TM Front Holder (Autodesk Fusion 360 design; units mm, degrees)
Autodesk Fusion 360 part; units mm, degrees
sketch "Sketch1" plane through (0, 0, 0) normal (0, 0, 1) x (1, 0, 0)
  line L0 (28.55, 26.275) -> (30.55, 26.275)
  line L1 (30.55, 26.275) -> (30.55, -30.825)
  line L2 (30.55, -30.825) -> (28.55, -30.825)
  line L3 (28.55, -30.825) -> (28.55, 26.275)
  line L4 (-28.55, -30.825) -> (-30.55, -30.825)
  line L5 (-28.55, 26.275) -> (-28.55, -30.825)
  line L6 (-30.55, -30.825) -> (-30.55, 26.275)
  line L7 (-30.55, 26.275) -> (-28.55, 26.275)
  line L8 (-30.55, 26.275) -> (30.55, 26.275)
  line L9 (30.55, 26.275) -> (30.55, 28.275)
  line L10 (30.55, 28.275) -> (-30.55, 28.275)
  line L11 (-30.55, 28.275) -> (-30.55, 26.275)
  dimension "d1" = 2
  dimension "d4" = 26.275
  dimension "d5" = 2
  dimension "d7" = 57.1
  dimension "d8" = 28.55
  dimension "d9" = 2
  dimension "d99" = 59.1
  constraint horizontal L0
  constraint vertical L1
  constraint horizontal L2
  constraint vertical L3
  constraint horizontal L7
  constraint vertical L5
  constraint horizontal L4
  constraint vertical L6
  constraint horizontal L2.end L4.start
  constraint horizontal L8
  constraint vertical L9
  constraint horizontal L10
  constraint vertical L11
  constraint vertical L0.end L9.end
  measures "d1" distance of L1 L3
  measures "d4" distance of origin L0
  measures "d5" distance of L5 L6
  measures "d7" distance of L3 L5
  measures "d8" distance of origin L5
  measures "d9" distance of L8 L10
  measures "d99" distance of L2 L10
extrude "Extrude1" add sketch "Sketch1" along normal blind 20
sketch "Sketch2" plane through (0, 0, 20) normal (0, 0, 1) x (-1, 0, 0)
  line L0 (-30.55, 30.825) -> (-30.55, -28.275)
  line L1 (-30.55, -28.275) -> (30.55, -28.275)
  line L2 (30.55, -28.275) -> (30.55, 30.825)
  line L3 (30.55, 30.825) -> (28.55, 30.825)
  line L4 (28.55, 30.825) -> (28.55, -26.275)
  line L5 (28.55, -26.275) -> (-28.55, -26.275)
  line L6 (-28.55, -26.275) -> (-28.55, 30.825)
  line L7 (-28.55, 30.825) -> (-30.55, 30.825)
  line L8 (-30.55, 30.825) -> (-40.55, 30.825)
  line L9 (-40.55, 30.825) -> (-40.55, 28.325)
  line L10 (-40.55, 28.325) -> (-30.55, 28.325)
  line L11 (-30.55, 28.325) -> (-30.55, 30.825)
  line L12 (30.55, 30.825) -> (40.55, 30.825)
  line L13 (40.55, 30.825) -> (40.55, 28.325)
  line L14 (40.55, 28.325) -> (30.55, 28.325)
  line L15 (30.55, 28.325) -> (30.55, 30.825)
  dimension "d12" = 2.5
  dimension "d13" = 10
  dimension "d14" = 2.5
  dimension "d15" = 10
  constraint horizontal L8
  constraint vertical L9
  constraint horizontal L10
  constraint vertical L11
  constraint coincident L0.start L7.end
  constraint horizontal L12
  constraint vertical L13
  constraint horizontal L14
  constraint vertical L15
  constraint coincident L2.end L3.start
  measures "d12" distance of L8 L10
  measures "d13" distance of L9 L11
  measures "d14" distance of L12 L14
  measures "d15" distance of L13 L15
extrude "Extrude2" add sketch "Sketch2" against normal blind 20 contours L0 L8 L9 L10 L11 | L2 L12 L13 L14 L15
sketch "Sketch5" plane through (0, 28.275, 0) normal (0, 1, 0) x (-1, 0, 0)
  line L0 (-30.55, 0) -> (30.55, 0)
  line L1 (30.55, 0) -> (30.55, 20)
  line L2 (30.55, 20) -> (-30.55, 20)
  line L3 (-30.55, 20) -> (-30.55, 0)
  line L4 (-20, 20) -> (20, 20)
  line L5 (20, 20) -> (20, 0)
  line L6 (20, 0) -> (-20, 0)
  line L7 (-20, 0) -> (-20, 20)
  dimension "d32" = 40
  dimension "d96" = 20
  constraint horizontal L4
  constraint vertical L5
  constraint horizontal L6
  constraint vertical L7
  constraint coincident L0 L5.end
  constraint coincident L2 L4.start
  measures "d32" distance of L5 L7
  measures "d96" distance of origin L7
extrude "Extrude4" add sketch "Sketch5" along normal blind 10 contours L0 L2 L4 L5 L6 L7
sketch "Sketch6" plane through (0, 0, 0) normal (0, 0, -1) x (1, 0, 0)
  line L0 (20, -38.275) -> (20, -28.275)
  line L1 (-30.55, -28.275) -> (-20, -28.275)
  line L2 (30.55, -28.275) -> (30.55, 28.325)
  line L3 (30.55, 28.325) -> (40.55, 28.325)
  line L4 (40.55, 30.825) -> (28.55, 30.825)
  line L5 (28.55, 30.825) -> (28.55, -26.275)
  line L6 (28.55, -26.275) -> (-28.55, -26.275)
  line L7 (-28.55, -26.275) -> (-28.55, 30.825)
  line L8 (-28.55, 30.825) -> (-40.55, 30.825)
  line L9 (-40.55, 28.325) -> (-30.55, 28.325)
  line L10 (-30.55, 28.325) -> (-30.55, -28.275)
  line L11 (-20, -28.275) -> (-20, -38.275)
  line L12 (-20, -38.275) -> (20, -38.275)
  line L13 (-28.55, -26.275) -> (-19.3, -26.275)
  line L14 (-19.3, -23.775) -> (-19.3, -22.025)
  line L15 (-24.3, -17.025) -> (-26.05, -17.025)
  line L16 (-28.55, -17.025) -> (-28.55, -26.275)
  line L17 (28.55, -26.275) -> (19.3, -26.275)
  line L18 (19.3, -23.775) -> (19.3, -22.025)
  line L19 (24.3, -17.025) -> (26.05, -17.025)
  line L20 (28.55, -17.025) -> (28.55, -26.275)
  arc A0 (-19.3, -22.025) -> (-24.3, -17.025) centre (-24.3, -22.025) ccw
  arc A1 (24.3, -17.025) -> (19.3, -22.025) centre (24.3, -22.025) ccw
  line L21 (28.55, -14.525) -> (28.55, -10)
  line L22 (-28.55, -14.525) -> (-28.55, -10)
  arc A2 (26.05, -17.025) -> (28.55, -14.525) centre (26.05, -14.525) ccw
  arc A3 (-28.55, -14.525) -> (-26.05, -17.025) centre (-26.05, -14.525) ccw
  line L23 (16.8, -26.275) -> (13, -26.275)
  line L24 (-16.8, -26.275) -> (-13, -26.275)
  arc A4 (16.8, -26.275) -> (19.3, -23.775) centre (16.8, -23.775) ccw
  arc A5 (-19.3, -23.775) -> (-16.8, -26.275) centre (-16.8, -23.775) ccw
  line L25 (20, -28.275) -> (30.55, -28.275)
  line L26 (-40.55, 30.825) -> (-40.55, 28.325)
  line L27 (40.55, 28.325) -> (40.55, 30.825)
  dimension "d38" = 9.25
  dimension "d39" = 9.25
  dimension "d40" = 9.25
  dimension "d41" = 9.25
  dimension "d42" = 5
  dimension "d43" = 5
  dimension "d44" = 2.5
  dimension "d45" = 2.5
  dimension "d46" = 2.5
  dimension "d47" = 2.5
  constraint horizontal L13
  constraint vertical L14
  constraint horizontal L15
  constraint vertical L16
  constraint coincident L6.end L7.start
  constraint horizontal L17
  constraint vertical L18
  constraint horizontal L19
  constraint vertical L20
  constraint coincident L5.end L6.start
  constraint tangent L15 A0
  constraint tangent L14 A0
  constraint tangent L19 A1
  constraint tangent L18 A1
  constraint coincident L5 L21.end
  constraint coincident L7 L22.end
  constraint coincident L20.start L19
  constraint coincident L20.start L21
  constraint tangent L19 A2
  constraint tangent L21 A2
  constraint coincident L16.start L22
  constraint coincident L16.start L15
  constraint tangent L22 A3
  constraint tangent L15 A3
  constraint coincident L6 L23.end
  constraint coincident L6 L24.end
  constraint coincident L17.end L23
  constraint coincident L17.end L18
  constraint tangent L23 A4
  constraint tangent L18 A4
  constraint coincident L13.end L24
  constraint coincident L13.end L14
  constraint tangent L24 A5
  constraint tangent L14 A5
  measures "d38" distance of L14 L16
  measures "d39" distance of L13 L15
  measures "d40" distance of L18 L20
  measures "d41" distance of L17 L19
  measures "d42" radius of A0
  measures "d43" radius of A1
  measures "d44" radius of A2
  measures "d45" radius of A3
  measures "d46" radius of A4
  measures "d47" radius of A5
extrude "Extrude5" add sketch "Sketch6" against normal blind 20 contours L5 L6 L17 L18 L19 L20 A1 A2 A4 | L6 L7 L13 L14 L15 L16 A0 A3 A5
sketch "Sketch7" plane through (0, 0, 20) normal (0, 0, 1) x (-1, 0, 0)
  line L0 (-30.55, -28.275) -> (-20, -28.275)
  line L1 (-20, -28.275) -> (20, -28.275)
  line L2 (30.55, -28.275) -> (30.55, 28.325)
  line L3 (30.55, 28.325) -> (40.55, 28.325)
  line L4 (40.55, 28.325) -> (40.55, 30.825)
  line L5 (40.55, 30.825) -> (28.55, 30.825)
  line L6 (28.55, 30.825) -> (28.55, -14.525)
  arc A0 (26.05, -17.025) -> (28.55, -14.525) centre (26.05, -14.525) ccw
  line L7 (26.05, -17.025) -> (24.3, -17.025)
  arc A1 (24.3, -17.025) -> (19.3, -22.025) centre (24.3, -22.025) ccw
  line L8 (19.3, -22.025) -> (19.3, -23.775)
  arc A2 (16.8, -26.275) -> (19.3, -23.775) centre (16.8, -23.775) ccw
  line L9 (16.8, -26.275) -> (-16.8, -26.275)
  arc A3 (-19.3, -23.775) -> (-16.8, -26.275) centre (-16.8, -23.775) ccw
  line L10 (-19.3, -23.775) -> (-19.3, -22.025)
  arc A4 (-19.3, -22.025) -> (-24.3, -17.025) centre (-24.3, -22.025) ccw
  line L11 (-24.3, -17.025) -> (-26.05, -17.025)
  arc A5 (-28.55, -14.525) -> (-26.05, -17.025) centre (-26.05, -14.525) ccw
  line L12 (-28.55, -14.525) -> (-28.55, 30.825)
  line L13 (-28.55, 30.825) -> (-40.55, 30.825)
  line L14 (-40.55, 30.825) -> (-40.55, 28.325)
  line L15 (-40.55, 28.325) -> (-30.55, 28.325)
  line L16 (-30.55, 28.325) -> (-30.55, -28.275)
  line L17 (20, -28.275) -> (30.55, -28.275)
  point P0 (24.05, -21.775)
  point P1 (-24.05, -21.775)
  dimension "d52" = 6.5
  dimension "d54" = 6.5
  constraint horizontal P0 P1
  measures "d52" distance of L2 P0
  measures "d54" distance of L16 P1
hole "Hole2" at (-24.05, 21.775, 20) at (24.05, 21.775, 20) direction (0, 0, -1) diameter 3 end through all
sketch "Sketch9" plane through (0, 38.275, 0) normal (0, 1, 0) x (-1, 0, 0)
  line L0 (-20, 0) -> (20, 0)
  line L1 (20, 20) -> (-20, 20)
  line L2 (-9.0392, 17) -> (9.0392, 17)
  line L3 (-9.0392, 3) -> (9.0392, 3)
  line L4 (-12, 15.1577) -> (-12, 4.8423)
  line L5 (12, 15.1577) -> (12, 4.8399)
  line L6 (-9.2786, 3.9389) -> (-0.2394, 8.8694)
  line L7 (-11.2606, 4.4033) -> (-1.8047, 9.5611)
  line L8 (-1.8047, 10.4389) -> (-11.2606, 15.5967)
  line L9 (11.2606, 15.5967) -> (1.7742, 10.4223)
  line L10 (-9.2786, 16.0611) -> (-0.2394, 11.1306)
  line L11 (0.2394, 11.1306) -> (9.2786, 16.0611)
  line L12 (0.2394, 8.8694) -> (9.2786, 3.9389)
  line L13 (1.7753, 9.5438) -> (11.2617, 4.4003)
  arc A0 (-11.2606, 15.5967) -> (-12, 15.1577) centre (-11.5, 15.1577) ccw
  arc A1 (-1.8047, 9.5611) -> (-1.8047, 10.4389) centre (-2.0442, 10) ccw
  arc A2 (-12, 4.8423) -> (-11.2606, 4.4033) centre (-11.5, 4.8423) ccw
  arc A3 (-9.2786, 3.9389) -> (-9.0392, 3) centre (-9.0392, 3.5) ccw
  arc A4 (0.2394, 8.8694) -> (-0.2394, 8.8694) centre (0, 8.4305) ccw
  arc A5 (9.0392, 3) -> (9.2786, 3.9389) centre (9.0392, 3.5) ccw
  arc A6 (11.2617, 4.4003) -> (12, 4.8399) centre (11.5, 4.8399) ccw
  arc A7 (1.7742, 10.4223) -> (1.7753, 9.5438) centre (2.0137, 9.9834) ccw
  arc A8 (12, 15.1577) -> (11.2606, 15.5967) centre (11.5, 15.1577) ccw
  arc A9 (9.2786, 16.0611) -> (9.0392, 17) centre (9.0392, 16.5) ccw
  arc A10 (-9.0392, 17) -> (-9.2786, 16.0611) centre (-9.0392, 16.5) ccw
  arc A11 (-0.2394, 11.1306) -> (0.2394, 11.1306) centre (0, 11.5695) ccw
  line L14 (20, 0) -> (20, 20)
  line L15 (-20, 20) -> (-20, 0)
  point P0 (11, 17)
  point P1 (12, 16)
  point P2 (0, 10)
  dimension "d60" = 11
  dimension "d61" = 6
  dimension "d62" = 0.5
  constraint horizontal L3
  constraint vertical L4
  constraint vertical L5
  constraint parallel L7 L9
  constraint tangent L4 A0
  constraint tangent L8 A0
  constraint tangent L8 A1
  constraint tangent L7 A1
  constraint equal A0 A1
  constraint tangent L4 A2
  constraint tangent L7 A2
  constraint equal A0 A2
  constraint tangent L3 A3
  constraint tangent L6 A3
  constraint equal A0 A3
  constraint tangent L12 A4
  constraint tangent L6 A4
  constraint equal A0 A4
  constraint tangent L12 A5
  constraint tangent L3 A5
  constraint equal A0 A5
  constraint tangent L13 A6
  constraint tangent L5 A6
  constraint equal A0 A6
  constraint tangent L9 A7
  constraint tangent L13 A7
  constraint equal A0 A7
  constraint coincident P1 L5
  constraint coincident P1 L9
  constraint tangent L5 A8
  constraint tangent L9 A8
  constraint equal A0 A8
  constraint coincident P0 L11
  constraint tangent L11 A9
  constraint tangent L2 A9
  constraint equal A0 A9
  constraint tangent L2 A10
  constraint tangent L10 A10
  constraint equal A0 A10
  constraint tangent L11 A11
  constraint tangent L10 A11
  constraint equal A0 A11
  measures "d60" horizontal distance of P0 P2
  measures "d61" vertical distance of P1 P2
  measures "d62" radius of A0
extrude "Extrude7" cut sketch "Sketch9" against normal blind 15 contours L2 L10 L11 A9 A10 A11 | L3 L6 L12 A3 A4 A5 | L4 L7 L8 A0 A1 A2 | L5 L9 L13 A6 A7 A8
sketch "Sketch10" plane through (-30.55, 0, 0) normal (-1, 0, 0) x (0, -1, 0)
  line L0 (-28.275, 0) -> (28.325, 0)
  line L1 (28.325, 0) -> (28.325, 20)
  line L2 (28.325, 20) -> (-28.275, 20)
  line L3 (-9.975, 15.25) -> (-9.975, 4.85)
  line L4 (14.525, 15.25) -> (14.525, 4.85)
  line L5 (-28.275, 20) -> (-28.275, 0)
  line L6 (-5.2906, 18) -> (9.8406, 18)
  line L7 (-5.2906, 2) -> (9.8406, 2)
  line L8 (-5.8274, 3.8437) -> (1.7382, 8.6576)
  line L9 (2.8118, 8.6576) -> (10.3774, 3.8437)
  line L10 (12.9967, 4.0009) -> (4.6396, 9.2009)
  line L11 (4.6396, 10.8991) -> (12.9967, 16.0991)
  line L12 (10.3774, 16.1563) -> (2.8118, 11.3424)
  line L13 (1.7382, 11.3424) -> (-5.8274, 16.1563)
  line L14 (-8.4467, 16.0991) -> (-0.0896, 10.8991)
  line L15 (-0.0896, 9.2009) -> (-8.4467, 4.0009)
  arc A0 (-8.4467, 16.0991) -> (-9.975, 15.25) centre (-8.975, 15.25) ccw
  arc A1 (-9.975, 4.85) -> (-8.4467, 4.0009) centre (-8.975, 4.85) ccw
  arc A2 (-0.0896, 9.2009) -> (-0.0896, 10.8991) centre (-0.6179, 10.05) ccw
  arc A3 (2.8118, 8.6576) -> (1.7382, 8.6576) centre (2.275, 7.8139) ccw
  arc A4 (9.8406, 2) -> (10.3774, 3.8437) centre (9.8406, 3) ccw
  arc A5 (-5.8274, 3.8437) -> (-5.2906, 2) centre (-5.2906, 3) ccw
  arc A6 (12.9967, 4.0009) -> (14.525, 4.85) centre (13.525, 4.85) ccw
  arc A7 (14.525, 15.25) -> (12.9967, 16.0991) centre (13.525, 15.25) ccw
  arc A8 (10.3774, 16.1563) -> (9.8406, 18) centre (9.8406, 17) ccw
  arc A9 (-5.2906, 18) -> (-5.8274, 16.1563) centre (-5.2906, 17) ccw
  arc A10 (1.7382, 11.3424) -> (2.8118, 11.3424) centre (2.275, 12.1861) ccw
  arc A11 (4.6396, 10.8991) -> (4.6396, 9.2009) centre (5.1679, 10.05) ccw
  line L16 (-28.275, 20) -> (-28.275, 0)
  point P0 (-9.975, 17.05)
  point P1 (-9.975, 3.05)
  point P2 (14.525, 17.05)
  point P3 (14.525, 3.05)
  point P4 (-8.725, 18)
  point P5 (13.275, 18)
  point P6 (-8.725, 2)
  point P7 (13.275, 2)
  point P8 (2.275, 10.05)
  dimension "d79" = 2
  dimension "d80" = 2
  dimension "d81" = 11
  dimension "d82" = 7
  dimension "d83" = 22
  dimension "d84" = 22
  dimension "d85" = 14
  dimension "d86" = 14
  dimension "d88" = 3.05
  dimension "d89" = 1
  dimension "d100" = 24.5
  dimension "d101" = 5.7857
  constraint perpendicular L2 L3
  constraint vertical L4
  constraint horizontal L6
  constraint perpendicular L3 L7
  constraint horizontal P0 P2
  constraint vertical P4 P6
  constraint coincident P0 L14
  constraint coincident P0 L3
  constraint tangent L14 A0
  constraint tangent L3 A0
  constraint coincident P1 L3
  constraint coincident P1 L15
  constraint tangent L3 A1
  constraint tangent L15 A1
  constraint equal A0 A1
  constraint tangent L15 A2
  constraint tangent L14 A2
  constraint equal A0 A2
  constraint tangent L8 A3
  constraint tangent L9 A3
  constraint equal A0 A3
  constraint coincident P7 L9
  constraint coincident P7 L7
  constraint tangent L9 A4
  constraint tangent L7 A4
  constraint equal A0 A4
  constraint coincident P6 L7
  constraint coincident P6 L8
  constraint tangent L7 A5
  constraint tangent L8 A5
  constraint equal A0 A5
  constraint coincident P3 L10
  constraint coincident P3 L4
  constraint tangent L10 A6
  constraint tangent L4 A6
  constraint equal A0 A6
  constraint coincident P2 L4
  constraint coincident P2 L11
  constraint tangent L4 A7
  constraint tangent L11 A7
  constraint equal A0 A7
  constraint coincident P5 L12
  constraint coincident P5 L6
  constraint tangent L12 A8
  constraint tangent L6 A8
  constraint equal A0 A8
  constraint coincident P4 L13
  constraint coincident P4 L6
  constraint tangent L13 A9
  constraint tangent L6 A9
  constraint equal A0 A9
  constraint tangent L13 A10
  constraint equal A0 A10
  constraint tangent L10 A11
  constraint tangent L11 A11
  constraint equal A0 A11
  constraint horizontal A0.centre A7.centre
  constraint horizontal A1.centre A6.centre
  constraint vertical A5.centre A9.centre
  constraint vertical A4.centre A8.centre
  constraint horizontal P8 A2.centre
  constraint vertical P8 A3.centre
  measures "d79" distance of L2 L6
  measures "d80" distance of L0 L7
  measures "d81" horizontal distance of P5 P8
  measures "d82" vertical distance of P2 P8
  measures "d83" distance of P4 P5
  measures "d84" distance of P6 P7
  measures "d85" distance of P2 P3
  measures "d86" distance of P0 P1
  measures "d88" distance of L0 P3
  measures "d89" radius of A0
  measures "d100" distance of L3 L4
  measures "d101" horizontal distance of A2.centre A11.centre
extrude "Extrude8" cut sketch "Sketch10" against normal blind 65 contours L3 L14 L15 A0 A1 A2 | L4 L10 L11 A6 A7 A11 | L6 L12 L13 A8 A9 A10 | L7 L8 L9 A3 A4 A5
extrude "Extrude9" cut 2 faces at (27.0333, 28.275, 6.6667) (-23.5167, 28.275, 13.3333) along direction (0, -1, 0) blind 1.55
extrude "Extrude10" cut 1 faces at (-17.3333, 38.275, 11.7192) along direction (0, -1, 0) blind 4.5
fillet "Fillet4" radius 2.5 6 edges at (-20, 26.725, 10) (-20, 33.775, 10) (-30.55, 26.725, 10) (20, 33.775, 10) (20, 26.725, 10) (30.55, 26.725, 10)
fillet "Fillet5" radius 2 2 edges at (-40.55, -29.575, 20) (40.55, -29.575, 20)
extrude "Extrude11" cut 2 faces at (-32.55, -30.825, 12.6667) (32.55, -30.825, 12.6667) along direction (0, 1, 0) blind 0.05
extrude "Extrude12" add 2 faces at (33.8833, -28.325, 12.6667) (-33.8833, -28.325, 12.6667) along direction (0, 1, 0) blind 7.55
sketch "Sketch11" plane through (0, -20.775, 0) normal (0, 1, 0) x (-1, 0, 0)
  arc A0 (-38.55, 20) -> (-40.55, 18) centre (-38.55, 18) ccw
  line L0 (-40.55, 18) -> (-40.55, 0)
  line L1 (-40.55, 0) -> (-30.55, 0)
  line L2 (-30.55, 0) -> (-30.55, 20)
  line L3 (-30.55, 20) -> (-38.55, 20)
  point P0 (-34.75, 10)
  point P1 (34.75, 10)
  dimension "d112" = 69.5
  dimension "d113" = 5.8
  dimension "d114" = 10
  constraint horizontal P0 P1
  measures "d112" distance of P0 P1
  measures "d113" distance of L0 P0
  measures "d114" distance of L3 P0
hole "Hole3" at (34.75, -20.775, 10) at (-34.75, -20.775, 10) direction (0, -1, 0) diameter 5.3 end through all counterbore diameter 10 counterbore depth 5
sketch "Sketch12" plane through (0, -20.775, 0) normal (0, 1, 0) x (-1, 0, 0)
  arc A0 (-30.55, 12.7129) -> (-30.55, 7.2871) centre (-34.75, 10) ccw
  line L0 (-30.55, 12.7129) -> (-30.55, 20)
  line L1 (-30.55, 20) -> (-38.55, 20)
  arc A1 (-38.55, 20) -> (-40.55, 18) centre (-38.55, 18) ccw
  line L2 (-40.55, 18) -> (-40.55, 0)
  line L3 (-40.55, 0) -> (-30.55, 0)
  line L4 (-30.55, 0) -> (-30.55, 7.2871)
  circle A2 centre (-34.75, 10) radius 5
  circle A3 centre (34.75, 10) radius 5
  dimension "d119" = 10
  dimension "d120" = 10
  dimension "d121" = 69.5
  constraint concentric A0 A2
  constraint horizontal A0.centre A3.centre
  measures "d119" diameter of A2
  measures "d120" diameter of A3
  measures "d121" distance of A0.centre A3.centre
extrude "Extrude13" cut sketch "Sketch12" along normal blind 7 contours A0 A2 | A3
equation "d4 = ( 52.55 / 2 ) * 1 mm"
equation "d8 = ( 57.1 / 2 ) * 1 mm"
equation "d88 = ( ( 20.1 - 14 ) / 2 ) * 1 mm"
equation "d99 = 57.55 mm + 1.55 mm"
equation "d110 = 10 mm - 2.45 mm"
